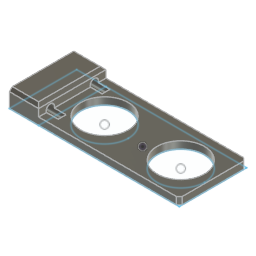
Ultrasonic-Sensor-Bracket-Vertical (Autodesk Fusion 360 design; units mm, degrees)
part number: 2026-04-13-02-21-18-182
Autodesk Fusion 360 part; units mm, degrees
sketch "Sketch1" plane through (0, 0, 0) normal (0, 0, 1) x (1, 0, 0)
  circle A0 centre (13, 0) radius 8.1
  circle A1 centre (-13, 0) radius 8.1
  line L0 (24, 11.5) -> (-24, 11.5)
  line L1 (-24, 11.5) -> (-24, -11.5)
  line L2 (-24, -11.5) -> (24, -11.5)
  line L3 (24, -11.5) -> (24, 11.5)
  line L4 (-24, 11.5) -> (-34, 11.5)
  line L5 (-34, 11.5) -> (-34, -11.5)
  line L6 (-34, -11.5) -> (-24, -11.5)
  dimension "d3" = 16.2
  dimension "d4" = 16.2
  constraint horizontal L0
  constraint perpendicular L0 L1
  constraint parallel L0 L2
  constraint parallel L1 L3
  constraint perpendicular L1 L4
  constraint perpendicular L0 L5
  constraint perpendicular L1 L6
  measures "d3" diameter of A0
  measures "d4" diameter of A1
extrude "Extrude1" add sketch "Sketch1" along normal blind 2 contours L0 L1 L2 L3 makes body 1
extrude "Extrude2" add sketch "Sketch1" along normal blind 2.5 separate body contours L0 L1 L2 L3 makes body 2
extrude "Extrude3" add sketch "Sketch1" along normal blind 6 contours L1 L4 L5 L6 bodies 1 2
sketch "Sketch3" plane through (-34, 0, 0) normal (-1, 0, 0) x (0, -1, 0)
  line L0 (-11.5, 0) -> (11.5, 0)
  line L1 (11.5, 0) -> (11.5, 6)
  line L2 (11.5, 6) -> (-11.5, 6)
  line L3 (-11.5, 6) -> (-11.5, 0)
  circle A0 centre (7.5, 3) radius 1.425
  circle A1 centre (-7.5, 3) radius 1.425
extrude "Extrude4" cut sketch "Sketch3" against normal blind 14 contours A0 | A1 bodies 1
chamfer "Chamfer1" distance 1 angle 45 5 edges at (-29, 11.5, 6) (-29, -11.5, 6) (-24, 0, 6) (24, 11.5, 1.25) (24, -11.5, 1.25) on bodies 1
